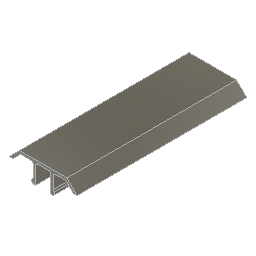
2020 Cover (Autodesk Fusion 360 design; units mm, degrees)
Autodesk Fusion 360 part; units mm, degrees
sketch "Sketch1" plane through (0, 0, 0) normal (0, 1, 0) x (1, 0, 0)
  line L0 (10, -10) -> (-10, -10)
  line L1 (-10, -10) -> (-10, 10)
  line L2 (-10, 10) -> (10, 10)
  line L3 (10, 10) -> (10, -10)
  line L4 (10, -10) -> (-10, 10) construction
  line L5 (-10, -10) -> (10, 10) construction
  line L6 (-10, -10) -> (10, -10)
  line L7 (10, -10) -> (10, -13)
  line L8 (10, -13) -> (-10, -13)
  line L9 (-10, -13) -> (-10, -10)
  line L10 (-3.75, -13) -> (-3.75, 10)
  line L11 (3.75, -13) -> (3.75, 10)
  line L12 (-2.95, -13) -> (-2.95, 10)
  line L13 (2.95, -13) -> (2.95, 10)
  line L14 (6, -13) -> (6, 10)
  line L15 (-6, 10) -> (-6, -13)
  line L16 (-10, -8) -> (10, -8)
  line L17 (-2.25, -13) -> (-2.25, 10)
  line L18 (2.25, -13) -> (2.25, 10)
  line L19 (10, -6.5) -> (-10, -6.5)
  line L20 (10, -12.2) -> (-10, -12.2)
  line L21 (6, -12.2) -> (9.182, -12.2) construction
  line L22 (6.3314, -13) -> (10.913, -13) construction
  line L23 (-6, -12.2) -> (-9.182, -12.2) construction
  line L24 (-6.3314, -13) -> (-10.9441, -13) construction
  line L25 (2.95, -8) -> (3.75, -7.2)
  line L26 (2.95, -8) -> (4.0607, -8) construction
  line L27 (2.95, -6.5) -> (3.75, -7.2)
  line L28 (-2.95, -8) -> (-3.75, -7.2)
  line L29 (-2.95, -8) -> (-4.0607, -8) construction
  line L30 (-2.95, -6.5) -> (-3.75, -7.2)
  line L31 (-10, -10) -> (-7, -13)
  line L32 (-10, -10) -> (-5.7574, -10) construction
  line L33 (-8.8686, -10) -> (-6.6686, -12.2)
  line L34 (10, -10) -> (7, -13)
  line L35 (10, -10) -> (5.7574, -10) construction
  line L36 (8.8686, -10) -> (6.6686, -12.2)
  line L37 (3.35, -8) -> (3.35, -6.5)
  line L38 (-3.35, -8) -> (-3.35, -6.5)
  dimension "d1" = 20
  dimension "d2" = 20
  dimension "d3" = 20
  dimension "d4" = 3
  dimension "d5" = 7.5
  dimension "d6" = 3.75
  dimension "d7" = 5.9
  dimension "d8" = 2.95
  dimension "d9" = 12
  dimension "d10" = 6
  dimension "d11" = 2
  dimension "d12" = 4.5
  dimension "d13" = 2.25
  dimension "d14" = 1.5
  dimension "d15" = 0.8
  dimension "d29" = 45
  dimension "d30" = 45
  dimension "d31" = 45
  dimension "d32" = 45
  dimension "d33" = 0.8
  dimension "d34" = 0.8
  dimension "d35" = 0.4
  dimension "d36" = 0.4
  constraint horizontal L0
  constraint perpendicular L0 L1
  constraint parallel L0 L2
  constraint parallel L1 L3
  constraint coincident L4 origin
  constraint coincident L5 origin
  constraint horizontal L6
  constraint vertical L7
  constraint horizontal L8
  constraint vertical L9
  constraint coincident L8 L10.start
  constraint coincident L2 L10.end
  constraint perpendicular L2 L10
  constraint coincident L8 L11.start
  constraint coincident L2 L11.end
  constraint perpendicular L2 L11
  constraint coincident L8 L12.start
  constraint coincident L2 L12.end
  constraint perpendicular L2 L12
  constraint coincident L8 L13.start
  constraint coincident L2 L13.end
  constraint perpendicular L2 L13
  constraint coincident L8 L14.start
  constraint coincident L2 L14.end
  constraint perpendicular L2 L14
  constraint coincident L2 L15.start
  constraint coincident L8 L15.end
  constraint perpendicular L8 L15
  constraint coincident L1 L16.start
  constraint coincident L3 L16.end
  constraint perpendicular L3 L16
  constraint coincident L8 L17.start
  constraint coincident L2 L17.end
  constraint perpendicular L2 L17
  constraint coincident L8 L18.start
  constraint coincident L2 L18.end
  constraint perpendicular L2 L18
  constraint coincident L3 L19.start
  constraint coincident L1 L19.end
  constraint perpendicular L1 L19
  constraint coincident L7 L20.start
  constraint coincident L9 L20.end
  constraint perpendicular L9 L20
  constraint horizontal L21
  constraint coincident L20 L21.start
  constraint coincident L14 L21.start
  constraint horizontal L22
  constraint coincident L8 L22.start
  constraint horizontal L23
  constraint coincident L20 L23.start
  constraint coincident L15 L23.start
  constraint horizontal L24
  constraint coincident L8 L24.start
  constraint horizontal L26
  constraint coincident L16 L25.start
  constraint coincident L13 L25.start
  constraint coincident L11 L25.end
  constraint coincident L19 L27.start
  constraint coincident L13 L27.start
  constraint horizontal L29
  constraint coincident L16 L28.start
  constraint coincident L12 L28.start
  constraint coincident L10 L28.end
  constraint coincident L19 L30.start
  constraint coincident L12 L30.start
  constraint horizontal L32
  constraint coincident L8 L31.end
  constraint coincident L0 L33.start
  constraint coincident L23 L33.end
  constraint parallel L31 L33
  constraint horizontal L35
  constraint coincident L8 L34.end
  constraint coincident L0 L36.start
  constraint coincident L20 L36.end
  constraint parallel L34 L36
  constraint coincident L16 L37.start
  constraint coincident L19 L37.end
  constraint perpendicular L19 L37
  constraint coincident L16 L38.start
  constraint coincident L19 L38.end
  constraint perpendicular L19 L38
  measures "d1" distance of L1.end L2.end
  measures "d2" distance of L0.end L1.end
  measures "d3" distance of L0.end L0.start
  measures "d4" distance of L0.end L8.end
  measures "d5" distance of L10 L11
  measures "d6" distance of origin L10
  measures "d7" distance of L12 L13
  measures "d8" distance of origin L12
  measures "d9" distance of L14 L15
  measures "d10" distance of origin L15
  measures "d11" distance of L0 L16
  measures "d12" distance of L17 L18
  measures "d13" distance of origin L17
  measures "d14" distance of L16 L19
  measures "d15" distance of L8 L20
  measures "d29" angle of L25 L26
  measures "d30" angle of L28 L29
  measures "d31" angle of L31 L32
  measures "d32" angle of L34 L35
  measures "d33" distance of L31 L33
  measures "d34" distance of L34 L36
  measures "d35" distance of L10 L38
  measures "d36" distance of L11 L37
extrude "Extrude1" add sketch "Sketch1" along normal blind 50 contours L0 L6 L20 L34 L36 | L8 L14 L20 L34 | L8 L11 L14 L20 | L0 L6 L13 L18 L20 | L0 L6 L13 L16 L18 | L8 L11 L13 L20 | L8 L13 L18 L20 | L13 L16 L18 L19 | L13 L25 L27 L37 | L0 L6 L12 L17 L20 | L0 L6 L12 L16 L17 | L8 L17 L18 L20 | L8 L12 L17 L20 | L12 L16 L17 L19 | L8 L10 L12 L20 | L12 L28 L30 L38 | L8 L10 L15 L20 | L0 L6 L20 L31 L33 | L8 L15 L20 L31
chamfer "Chamfer5" distance 0.5 angle 45 4 edges at (-2.25, 25, 12.2) (-2.95, 25, 12.2) (2.25, 25, 12.2) (2.95, 25, 12.2)
